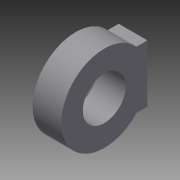
# Autodesk Inventor part: Wall Hoop
Saved by Autodesk Inventor 2015 (Build 190159000, 159)
## iProperties
Created: 2016-12-01
Part Number: Wall Hoop
Material: Generic
Document SubType Name: Modeling
Designer: Simms
Density: 1 g/cm^3
Appearance: Default
Author: Simms
Autodesk Inventor part; units mm, degrees
ref_plane "YZ Plane" through (0, 0, 0) normal (1, 0, 0) x (0, 1, 0)
ref_plane "XZ Plane" through (0, 0, 0) normal (0, 1, 0) x (-1, 0, 0)
ref_plane "XY Plane" through (0, 0, 0) normal (0, 0, 1) x (1, 0, 0)
sketch "Sketch1" plane through (0, 0, 0) normal (0, 0, 1) x (1, 0, 0)
  line L0 (0, 0) -> (6.35, 0)
  line L1 (6.35, 0) -> (6.35, 12.7)
  line L2 (6.35, 12.7) -> (0, 12.7)
  line L3 (0, 12.7) -> (0, 0)
  dimension "d0" = 6.35
  dimension "d1" = 12.7
  constraints: 8 end point, 2 parallel, 1 horizontal, 1 perpendicular
  measures "d0" distance of L2.end L1.end
  measures "d1" distance of L1.end L0.end
extrude "Extrusion1" add sketch "Sketch1" along normal blind 3.175
sketch "Sketch2" plane through (6.35, 0, 0) normal (1, 0, 0) x (0, 0, -1)
  circle A0 centre (-9.525, 6.35) radius 9.525
  line L0 (0, 0) -> (0, 12.7) projected
  circle A1 centre (-9.525, 6.35) radius 4.7625
  dimension "d4" = 9.525
  constraints: 2 centre point, 1 coincident, 1 tangent
  measures "d4" diameter of A1
extrude "Extrusion2" add sketch "Sketch2" against normal blind 6.35
body "Solid1"
